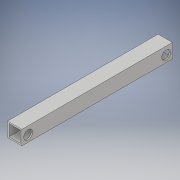
# Autodesk Inventor part: push bar
Saved by Autodesk Inventor 2018 (Build 220112000, 112)
## iProperties
Created: 2019-01-18
Part Number: push bar
Material: Generic
Document SubType Name: Modeling
Designer: s-4008082
Density: 1 g/cm^3
Appearance: Default
Author: s-4008082
Autodesk Inventor part; units mm, degrees
ref_plane "YZ Plane" through (0, 0, 0) normal (1, 0, 0) x (0, 1, 0)
ref_plane "XZ Plane" through (0, 0, 0) normal (0, 1, 0) x (-1, 0, 0)
ref_plane "XY Plane" through (0, 0, 0) normal (0, 0, 1) x (1, 0, 0)
sketch "Sketch1" plane through (0, 0, 0) normal (0, 0, 1) x (1, 0, 0)
  line L0 (12.7, -12.7) -> (-12.7, -12.7)
  line L1 (-12.7, -12.7) -> (-12.7, 12.7)
  line L2 (-12.7, 12.7) -> (12.7, 12.7)
  line L3 (12.7, 12.7) -> (12.7, -12.7)
  line L4 (12.7, -12.7) -> (-12.7, 12.7) construction
  line L5 (-12.7, -12.7) -> (12.7, 12.7) construction
  line L6 (10.16, 10.16) -> (-10.16, 10.16)
  line L7 (-10.16, 10.16) -> (-10.16, -10.16)
  line L8 (-10.16, -10.16) -> (10.16, -10.16)
  line L9 (10.16, -10.16) -> (10.16, 10.16)
  line L10 (10.16, 10.16) -> (-10.16, -10.16) construction
  line L11 (-10.16, 10.16) -> (10.16, -10.16) construction
  point P0 (0, 0)
  dimension "d0" = 25.4
  dimension "d1" = 25.4
  dimension "d2" = 2.54
  dimension "d3" = 2.54
  constraints: 24 end point, 4 midpoint, 4 parallel, 2 horizontal, 2 perpendicular
  measures "d0" distance of L1.end L2.end
  measures "d1" distance of L0.end L1.end
  measures "d2" distance between parallel lines of L1 L7
  measures "d3" distance between parallel lines of L0 L8
extrude "Extrusion1" add sketch "Sketch1" along normal blind 266.7
sketch "Sketch2" plane through (12.7, -12.7, 0) normal (1, 0, 0) x (0, 0, -1)
  circle A0 centre (-11.0998, 11.6207) radius 7.9375
  circle A1 centre (-255.6002, 11.6207) radius 7.9375
  line L0 (0, 25.4) -> (0, 0) projected
  line L1 (-266.7, 0) -> (-266.7, 25.4) projected
  point P0 (0, 12.7)
  dimension "d6" = 244.5004
  dimension "d7" = 15.875
  dimension "d8" = 15.875
  dimension "d9" = 11.0998
  dimension "d10" = 11.0998
  constraints: 2 centre point
  measures "d6" distance of A0.centre A1.centre
  measures "d7" diameter of A0
  measures "d8" diameter of A1
  measures "d9" distance from line of L0 A0.centre
  measures "d10" distance from line of L1 A1.centre
extrude "Extrusion2" cut sketch "Sketch2" against normal blind 2.54
equation "\"d3\" = d2"
equation "\"d8\" = d7"
body "Solid1"
